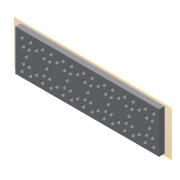
# Autodesk Inventor part: phone mount base
Saved by Autodesk Inventor 2018 (Build 220112000, 112)
## iProperties
Created: 2019-02-12
Part Number: phone mount base
Material: Generic
Document SubType Name: Modeling
Designer: ball
Density: 1 g/cm^3
Appearance: Default
Author: ball
Autodesk Inventor part; units mm, degrees
ref_plane "YZ Plane" through (0, 0, 0) normal (1, 0, 0) x (0, 1, 0)
ref_plane "XZ Plane" through (0, 0, 0) normal (0, 1, 0) x (-1, 0, 0)
ref_plane "XY Plane" through (0, 0, 0) normal (0, 0, 1) x (1, 0, 0)
ref_plane "Work Plane1" through (0, 0, 0) normal (0, 0, 1) x (1, 0, 0)
sketch "Sketch1" plane through (0, 0, 0) normal (0, 0, 1) x (1, 0, 0)
  line L0 (-66.675, -19.05) -> (66.675, -19.05) projected
  line L1 (66.675, -19.05) -> (66.675, 19.05) projected
  line L2 (66.675, 19.05) -> (-66.675, 19.05) projected
  line L3 (-66.675, 19.05) -> (-66.675, -19.05) projected
  circle A0 centre (61.0954, -13.4704) radius 1.778 construction
  circle A1 centre (59.7602, -6.9148) radius 1.778 construction
  circle A2 centre (57.15, 0) radius 2.032 construction
  circle A3 centre (54.5398, -6.9148) radius 1.778 construction
  circle A4 centre (53.2046, -13.4704) radius 1.778 construction
  circle A5 centre (54.5398, 6.9148) radius 1.778 construction
  circle A6 centre (53.2046, 13.4704) radius 1.778 construction
  circle A7 centre (59.7602, 6.9148) radius 1.778 construction
  circle A8 centre (61.0954, 13.4704) radius 1.778 construction
  circle A9 centre (47.625, 9.779) radius 1.778 construction
  circle A10 centre (47.625, -9.779) radius 1.778 construction
  circle A11 centre (61.0954, -13.4704) radius 1.9685
  circle A12 centre (59.7602, -6.9148) radius 1.9685
  circle A13 centre (53.2046, -13.4704) radius 1.9685
  circle A14 centre (54.5398, -6.9148) radius 1.905
  circle A15 centre (57.15, 0) radius 1.9685
  circle A16 centre (59.7602, 6.9148) radius 1.9685
  circle A17 centre (54.5398, 6.9148) radius 1.9685
  circle A18 centre (61.0954, 13.4704) radius 1.9685
  circle A19 centre (53.2046, 13.4704) radius 1.9685
  circle A20 centre (47.625, 9.779) radius 1.9685
  circle A21 centre (47.625, -9.779) radius 1.9685
  circle A22 centre (34.1546, -13.4704) radius 1.778 construction
  point P0 (0, 0)
  dimension "d0" = 3.937
  dimension "d1" = 3.937
  dimension "d2" = 3.937
  dimension "d3" = 3.81
  dimension "d4" = 3.937
  dimension "d5" = 3.937
  dimension "d6" = 3.937
  dimension "d7" = 3.937
  dimension "d8" = 3.937
  dimension "d9" = 3.937
  dimension "d10" = 3.937
  constraints: 11 centre point, 11 coincident
  measures "d0" diameter of A11
  measures "d1" diameter of A12
  measures "d2" diameter of A13
  measures "d3" diameter of A14
  measures "d4" diameter of A15
  measures "d5" diameter of A16
  measures "d6" diameter of A17
  measures "d7" diameter of A18
  measures "d8" diameter of A19
  measures "d9" diameter of A20
  measures "d10" diameter of A21
extrude "Extrusion1" add sketch "Sketch1" along normal blind 5.08
body "Solid1"
